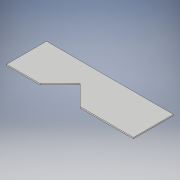
# Autodesk Inventor part: motorMountAndRopeGuide
Saved by Autodesk Inventor 2017 (Build 210142000, 142)
## iProperties
Created: 2017-02-02
Part Number: motorMountAndRopeGuide
Material: Generic
Document SubType Name: Sheet Metal
Designer: kingb
Density: 1 g/cm^3
Sheet Metal Rule: Default
Appearance: Default
Author: kingb
Autodesk Inventor part; units mm, degrees
ref_plane "YZ Plane" through (0, 0, 0) normal (1, 0, 0) x (0, 1, 0)
ref_plane "XZ Plane" through (0, 0, 0) normal (0, 1, 0) x (-1, 0, 0)
ref_plane "XY Plane" through (0, 0, 0) normal (0, 0, 1) x (1, 0, 0)
sketch "Sketch1" plane through (0, 0, 0) normal (0, 1, 0) x (-1, 0, 0)
  line L0 (-322.58, 0) -> (-322.58, -101.6)
  line L1 (-322.58, -101.6) -> (0, -101.6)
  line L2 (0, -101.6) -> (0, 0)
  line L3 (-186.69, 0) -> (-135.89, -50.8)
  line L4 (-135.89, -50.8) -> (-85.09, 0)
  line L5 (0, 0) -> (-85.09, 0)
  line L6 (-186.69, 0) -> (-322.58, 0)
  dimension "d0" = 322.58
  dimension "d1" = 101.6
  dimension "d5" = 50.8
  dimension "d7" = 85.09
  dimension "d8" = 135
  dimension "d9" = 135
  dimension "d10" = 0
  measures "d0" distance of L1.end L0.end
  measures "d1" distance of L0.end L0.start
  measures "d5" distance from line of L1 L3.end
  measures "d7" distance of L2.end L4.end
  measures "d8" angle of L5 L4
  measures "d9" angle of L6 L3
  measures "d10" vertical distance of L0.start L4.end
extrude "Plate1" add sketch "Sketch1" along normal blind 3.048
equation "\"BendRadius\" = Thickness"
equation "\"BendReliefWidth\" = Thickness"
equation "\"BendReliefDepth\" = 0.5 * Thickness"
equation "\"CornerReliefSize\" = 4 * Thickness"
equation "\"MinimumRemnant\" = 2 * Thickness"
equation "\"TransitionRadius\" = BendRadius"
equation "\"JacobiRadiusSize\" = BendRadius"
equation "\"GapSize\" = Thickness"
equation "\"d2\" = BendRadius"
equation "\"Thickness\" = 3.048"
body "Solid1"
